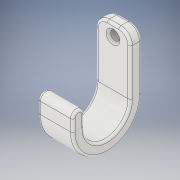
# Autodesk Inventor part: curved_single_hook
Saved by Autodesk Inventor 2019 (Build 230136000, 136)
## iProperties
Created: 2019-02-20
Part Number: curved_single_hook
Material: PET Plastic
Document SubType Name: Modeling
Designer: jmc
Density: 1.541 g/cm^3
Appearance: White
Author: jmc
## iProperties of the stored document curved_single_hook_3DPrint.ipt
Created: 2019-02-20
Part Number: curved_single_hook_3DPrint
Material: Generic
Document SubType Name: Modeling
Designer: jmc
Density: 1 g/cm^3
Appearance: Default
Author: jmc
Autodesk Inventor part; units mm, degrees
ref_plane "YZ Plane" through (0, 0, 0) normal (1, 0, 0) x (0, 1, 0)
ref_plane "XZ Plane" through (0, 0, 0) normal (0, 1, 0) x (-1, 0, 0)
ref_plane "XY Plane" through (0, 0, 0) normal (0, 0, 1) x (1, 0, 0)
sketch "Sketch1" plane through (0, 0, 0) normal (0, 0, 1) x (1, 0, 0)
  line L0 (-2.5, 12.5) -> (2.5, 12.5)
  line L1 (7.5, 7.5) -> (7.5, -12.5)
  line L2 (7.5, -12.5) -> (-7.5, -12.5)
  line L3 (-7.5, -12.5) -> (-7.5, 7.5)
  line L4 (-7.5, 12.5) -> (7.5, -12.5) construction
  line L5 (7.5, 12.5) -> (-7.5, -12.5) construction
  arc A0 (-2.5, 12.5) -> (-7.5, 7.5) centre (-2.5, 7.5) ccw
  arc A1 (7.5, 7.5) -> (2.5, 12.5) centre (2.5, 7.5) ccw
  circle A2 centre (0, 7.5) radius 1.5
  point P0 (0, 0)
  dimension "d0" = 15
  dimension "d3" = 5
  dimension "d4" = 3
  dimension "d5" = 5
  dimension "HOOK_HEIGHT" = 20
  constraints: 12 end point, 4 point on circle, 4 point on line, 4 tangent, 3 centre point, 2 midpoint, 2 parallel, 1 equal radius, 1 horizontal, 1 perpendicular
  measures "d0" distance of L1.end L2.end
  measures "d3" radius of A0
  measures "d4" diameter of A2
  measures "d5" distance from line of L0 A2.centre
  measures "HOOK_HEIGHT" distance of L2.end L3.end
extrude "Extrusion2" add sketch "Sketch1" along normal blind 5
sketch "Sketch2" plane through (0, 0, 5) normal (0, 0, 1) x (1, 0, 0)
  circle A0 centre (0, 7.5) radius 1.5 projected
  point P0 (0, 0)
  constraints: 1 coincident
hole "Hole1" at (0, 7.5, 5) direction (0, 0, -1) diameter 4 end through all countersink diameter 6 countersink angle 90
sketch "Sketch3" plane through (-7.5, -12.5, 0) normal (-1, 0, 0) x (0, 0, 1)
  line L0 (0, 0) -> (5, 0)
  line L1 (2.5, 0) -> (2.5, -6.8079) construction
  arc A0 (0, 0) -> (30, 0) centre (15, 0) ccw
  line L2 (5, 20) -> (5, 0) construction
  line L3 (0, 20) -> (0, 0) construction
  arc A1 (5, 0) -> (25, 0) centre (15, 0) ccw
  line L4 (25, 0) -> (25, 5)
  line L5 (30, 5) -> (30, 0)
  arc A2 (30, 5) -> (25, 5) centre (27.5, 5) ccw
  point P0 (0, 12.5)
  dimension "HOOK_RADIUS" = 30
  dimension "d16" = 5
  dimension "HOOK_LEN" = 5
  dimension "d18" = 5
  constraints: 8 end point, 6 point on circle, 3 centre point, 3 tangent, 2 vertical, 1 coincident, 1 midpoint
  measures "HOOK_RADIUS" diameter of A0
  measures "d16" radial gap between concentric circles of A0 A1
  measures "HOOK_LEN" distance of L4.start L4.end
  measures "d18" diameter of A2
extrude "Extrusion3" add sketch "Sketch3" against normal up to surface (15 mm away)
fillet "Fillet1" radius 1 18 edges at (7.5, -2.5, 5) (6.0355, 11.0355, 5) (0, 12.5, 5) (-6.0355, 11.0355, 5) (-7.5, -2.5, 5) (-7.5, -22.5, 15) (-7.5, -10, 25) (-7.5, -5, 27.5) (-7.5, -10, 30) (-7.5, -27.5, 15) (-7.5, -2.5, 0) (-6.0355, 11.0355, 0) (0, 12.5, 0) (6.0355, 11.0355, 0) (7.5, -2.5, 0) (7.5, -10, 30) (7.5, -5, 27.5) (7.5, -10, 25)
body "Solid2"
